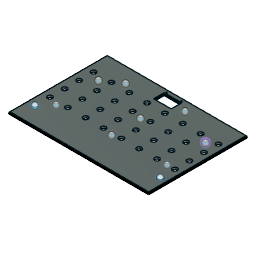
SQ-80_Lid2 (Autodesk Fusion 360 design; units mm, degrees)
part number: 2026-07-01-17-07-32-906
Autodesk Fusion 360 part; units mm, degrees
sketch "Sketch1" plane through (0, 0, 0) normal (0, 0, 1) x (1, 0, 0)
  line L0 (0, 0) -> (225, 0)
  line L1 (225, 0) -> (225, 158.6)
  line L2 (225, 158.6) -> (0, 158.6)
  line L3 (0, 158.6) -> (0, 0)
  dimension "d1" = 158.6
  dimension "d2" = 225
  constraint horizontal L0
  constraint vertical L1
  constraint horizontal L2
  constraint vertical L3
  constraint coincident L0.start L3.end
  measures "d1" distance of L0.end L1.end
  measures "d2" distance of L1.end L2.end
extrude "Extrude1" add sketch "Sketch1" along normal blind 3
sketch "Sketch2" plane through (0, 0, 3) normal (0, 0, 1) x (-1, 0, 0)
  line L0 (0, -158.6) -> (0, 0)
  line L1 (0, 0) -> (-225, 0)
  line L2 (-225, 0) -> (-225, -158.6)
  line L3 (-225, -158.6) -> (0, -158.6)
  circle A0 centre (-13, -123.6) radius 3.25
  dimension "d5" = 13
  dimension "d6" = 35
  dimension "d7" = 6.5
  measures "d5" distance of L0 A0.centre
  measures "d6" distance of L3 A0.centre
  measures "d7" diameter of A0
hole "Hole1" at (13, 123.6, 3) direction (0, 0, -1) diameter 7.75 end through all
pattern_linear "R-Pattern4" count 4 spacing 23.3333 along (0, -1, 0) count 8 spacing 28.6429 along (1, 0, 0) of "Hole1"
sketch "MountingPostsSketch" plane through (0, 0, 0) normal (0, 0, 1) x (1, 0, 0)
  circle A0 centre (25.79, 118.58) radius 4
  circle A1 centre (25.79, 50.49) radius 4
  circle A2 centre (51.81, 136.5) radius 4
  circle A3 centre (112.44, 99.27) radius 4
  circle A4 centre (112.44, 53.03) radius 4
  circle A5 centre (138.38, 144.98) radius 4
  circle A6 centre (198.31, 117.8) radius 4
  circle A7 centre (198.31, 56.27) radius 4
  dimension "d47" = 8
  dimension "d48" = 8
  dimension "d50" = 8
  dimension "d51" = 8
  dimension "d52" = 8
  dimension "d53" = 8
  dimension "d54" = 8
  dimension "d55" = 8
  measures "d47" diameter of A5
  measures "d48" diameter of A3
  measures "d50" diameter of A4
  measures "d51" diameter of A1
  measures "d52" diameter of A0
  measures "d53" diameter of A2
  measures "d54" diameter of A7
  measures "d55" diameter of A6
extrude "Extrude2" add sketch "MountingPostsSketch" against normal blind 9
sketch "M3HolesSketch" plane through (0, 0, 0) normal (0, 0, 1) x (1, 0, 0)
  circle A0 centre (25.79, 118.58) radius 1.6
  circle A1 centre (25.79, 50.49) radius 1.6
  circle A2 centre (51.91, 136) radius 1.6
  circle A3 centre (112.54, 99.27) radius 1.6
  circle A4 centre (112.44, 53.03) radius 1.6
  circle A5 centre (138.38, 144.98) radius 1.6
  circle A6 centre (198.31, 117.8) radius 1.6
  circle A7 centre (198.31, 56.27) radius 1.6
  circle A8 centre (198.31, 117.8) radius 4
  dimension "d49" = 8
  measures "d49" diameter of A8
ref_plane "WorkPlane1" through (0, 0, 2) normal (0, 0, 1) x (1, 0, 0)
sketch "OLED_Opening_Sketch" plane through (0, 0, 2) normal (0, 0, 1) x (1, 0, 0)
  line L0 (99.5, 135.6) -> (125.5, 135.6)
  line L1 (125.5, 135.6) -> (125.5, 150.35)
  line L2 (125.5, 150.35) -> (99.5, 150.35)
  line L3 (99.5, 150.35) -> (99.5, 135.6)
extrude "Extrude4" cut sketch "OLED_Opening_Sketch" along normal through all and the other way through all
ref_plane "WorkPlane2" through (0, 0, 2) normal (0, 0, 1) x (1, 0, 0)
sketch "MountingHoles_Sketch" plane through (0, 0, 2) normal (0, 0, 1) x (1, 0, 0)
  circle A0 centre (100.5, 153.1) radius 1.3
  circle A1 centre (124.5, 153.1) radius 1.3
  dimension "d56" = 2.6
  dimension "d57" = 2.6
  measures "d56" diameter of A0
  measures "d57" diameter of A1
extrude "Extrude5" cut sketch "MountingHoles_Sketch" along normal blind 15 and the other way blind 3
sketch "Sketch7" plane through (0, 0, 0) normal (0, 0, -1) x (1, 0, 0)
  line L0 (125.5, -150.35) -> (99.5, -150.35)
  line L1 (99.5, -150.35) -> (99.5, -135.6)
  line L2 (99.5, -135.6) -> (125.5, -135.6)
  line L3 (125.5, -135.6) -> (125.5, -150.35)
  circle A0 centre (213.5003, -76.9334) radius 3.875
  circle A1 centre (213.5003, -123.6) radius 3.875
  circle A2 centre (184.8574, -76.9334) radius 3.875
  circle A3 centre (184.8574, -123.6) radius 3.875
  circle A4 centre (156.2145, -76.9334) radius 3.875
  circle A5 centre (156.2145, -123.6) radius 3.875
  circle A6 centre (127.5716, -76.9334) radius 3.875
  circle A7 centre (127.5716, -123.6) radius 3.875
  circle A8 centre (98.9287, -76.9334) radius 3.875
  circle A9 centre (98.9287, -123.6) radius 3.875
  circle A10 centre (70.2858, -76.9334) radius 3.875
  circle A11 centre (70.2858, -123.6) radius 3.875
  line L4 (0, 0) -> (0, -158.6)
  line L5 (0, -158.6) -> (225, -158.6)
  line L6 (225, -158.6) -> (225, 0)
  line L7 (225, 0) -> (0, 0)
  circle A12 centre (13, -123.6) radius 3.875
  circle A13 centre (13, -100.2667) radius 3.875
  circle A14 centre (13, -76.9334) radius 3.875
  circle A15 centre (13, -53.6001) radius 3.875
  circle A16 centre (41.6429, -123.6) radius 3.875
  circle A17 centre (41.6429, -100.2667) radius 3.875
  circle A18 centre (41.6429, -76.9334) radius 3.875
  circle A19 centre (41.6429, -53.6001) radius 3.875
  circle A20 centre (70.2858, -100.2667) radius 3.875
  circle A21 centre (70.2858, -53.6001) radius 3.875
  circle A22 centre (98.9287, -100.2667) radius 3.875
  circle A23 centre (98.9287, -53.6001) radius 3.875
  circle A24 centre (127.5716, -100.2667) radius 3.875
  circle A25 centre (127.5716, -53.6001) radius 3.875
  circle A26 centre (156.2145, -100.2667) radius 3.875
  circle A27 centre (156.2145, -53.6001) radius 3.875
  circle A28 centre (184.8574, -100.2667) radius 3.875
  circle A29 centre (184.8574, -53.6001) radius 3.875
  circle A30 centre (213.5003, -100.2667) radius 3.875
  circle A31 centre (213.5003, -53.6001) radius 3.875
  line L8 (118.5096, -127.6004) -> (106.547, -127.6004)
  line L9 (106.547, -127.6004) -> (106.547, -126.0574)
  line L10 (106.547, -126.0574) -> (118.5096, -126.0574)
  line L11 (118.5096, -126.0574) -> (118.5096, -127.6004)
  circle A32 centre (138.38, -144.98) radius 4
  circle A33 centre (51.81, -136.5) radius 4
  circle A34 centre (112.44, -99.27) radius 4
  circle A35 centre (198.31, -117.8) radius 4
  circle A36 centre (112.44, -53.03) radius 4
  circle A37 centre (25.79, -50.49) radius 4
  circle A38 centre (25.79, -118.58) radius 4
  circle A39 centre (198.31, -56.27) radius 4
  circle A40 centre (124.5, -153.1) radius 1.3
  circle A41 centre (100.5, -153.1) radius 1.3
  constraint horizontal L8
  constraint vertical L9
  constraint horizontal L10
  constraint vertical L11
extrude "Extrude6" add sketch "Sketch7" along normal blind 3 contours L8 L9 L10 L11
sketch "Sketch8" plane through (0, 0, -3) normal (0, 0, -1) x (1, 0, 0)
  line L0 (118.5096, -126.0574) -> (106.547, -126.0574)
  line L1 (106.547, -126.0574) -> (106.547, -127.6004)
  line L2 (106.547, -127.6004) -> (118.5096, -127.6004)
  line L3 (118.5096, -127.6004) -> (118.5096, -126.0574)
  line L4 (118.5096, -126.0574) -> (106.4856, -126.0574)
  line L5 (106.4856, -126.0574) -> (106.4856, -129.1746)
  line L6 (106.4856, -129.1746) -> (118.5096, -129.1746)
  line L7 (118.5096, -129.1746) -> (118.5096, -126.0574)
  constraint horizontal L4
  constraint vertical L5
  constraint horizontal L6
  constraint vertical L7
  constraint coincident L0.start L3.end
extrude "Extrude3" cut sketch "M3HolesSketch" against normal blind 9 contours A0 | A1 | A2 | A3 | A4 | A5 | A6 | A7
extrude "Extrude7" add sketch "Sketch8" along normal blind 1.5
chamfer "Chamfer1" distance 1 angle 45 4 edges at (225, 79.3, 3) (112.5, 158.6, 3) (0, 79.3, 3) (112.5, 0, 3)
chamfer "Chamfer2" distance 1 angle 45 4 edges at (112.5, 135.6, 3) (99.5, 142.975, 3) (112.5, 150.35, 3) (125.5, 142.975, 3)
sketch "Sketch9" plane through (0, 0, 3) normal (0, 0, 1) x (-1, 0, 0)
  line L0 (-1, -157.6) -> (-1, -1)
  line L1 (-1, -1) -> (-224, -1)
  line L2 (-224, -1) -> (-224, -157.6)
  line L3 (-224, -157.6) -> (-1, -157.6)
  circle A0 centre (-213.5003, -76.9334) radius 3.875
  circle A1 centre (-213.5003, -123.6) radius 3.875
  circle A2 centre (-184.8574, -76.9334) radius 3.875
  circle A3 centre (-184.8574, -123.6) radius 3.875
  circle A4 centre (-156.2145, -76.9334) radius 3.875
  circle A5 centre (-156.2145, -123.6) radius 3.875
  circle A6 centre (-127.5716, -76.9334) radius 3.875
  circle A7 centre (-127.5716, -123.6) radius 3.875
  circle A8 centre (-98.9287, -76.9334) radius 3.875
  circle A9 centre (-98.9287, -123.6) radius 3.875
  circle A10 centre (-70.2858, -76.9334) radius 3.875
  circle A11 centre (-70.2858, -123.6) radius 3.875
  circle A12 centre (-13, -123.6) radius 3.875
  circle A13 centre (-13, -100.2667) radius 3.875
  circle A14 centre (-13, -76.9334) radius 3.875
  circle A15 centre (-13, -53.6001) radius 3.875
  circle A16 centre (-41.6429, -123.6) radius 3.875
  circle A17 centre (-41.6429, -100.2667) radius 3.875
  circle A18 centre (-41.6429, -76.9334) radius 3.875
  circle A19 centre (-41.6429, -53.6001) radius 3.875
  circle A20 centre (-70.2858, -100.2667) radius 3.875
  circle A21 centre (-70.2858, -53.6001) radius 3.875
  circle A22 centre (-98.9287, -100.2667) radius 3.875
  circle A23 centre (-98.9287, -53.6001) radius 3.875
  circle A24 centre (-127.5716, -100.2667) radius 3.875
  circle A25 centre (-127.5716, -53.6001) radius 3.875
  circle A26 centre (-156.2145, -100.2667) radius 3.875
  circle A27 centre (-156.2145, -53.6001) radius 3.875
  circle A28 centre (-184.8574, -100.2667) radius 3.875
  circle A29 centre (-184.8574, -53.6001) radius 3.875
  circle A30 centre (-213.5003, -100.2667) radius 3.875
  circle A31 centre (-213.5003, -53.6001) radius 3.875
  circle A32 centre (-124.5, -153.1) radius 1.3
  circle A33 centre (-100.5, -153.1) radius 1.3
  line L4 (-126.5, -134.6) -> (-98.5, -134.6)
  line L5 (-98.5, -134.6) -> (-98.5, -151.35)
  line L6 (-98.5, -151.35) -> (-126.5, -151.35)
  line L7 (-126.5, -151.35) -> (-126.5, -134.6)
  circle A34 centre (-213.6, -30) radius 4
  circle A35 centre (-12.6309, -29.642) radius 4
  dimension "d58" = 8
  dimension "d62" = 8
  measures "d58" diameter of A34
  measures "d62" diameter of A35
hole "Hole2" at (213.6, 30, 3) direction (0, 0, -1) diameter 8 depth 3 tip angle 118
hole "Hole3" at (12.6309, 29.642, 3) direction (0, 0, -1) diameter 7 depth 3 tip angle 118
equation "d22 = -( 9 mm )"
equation "d24 = -( 9 mm )"
